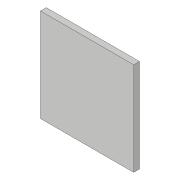
# Autodesk Inventor part: upper part of cappinng system
Saved by Autodesk Inventor 2019 (Build 230136000, 136)
## iProperties
Created: 2019-10-12
Part Number: upper part of cappinng system
Material: Generic
Document SubType Name: Modeling
Designer: Admin
Density: 1 g/cm^3
Appearance: Default
Author: Admin
Autodesk Inventor part; units mm, degrees
ref_plane "YZ Plane" through (0, 0, 0) normal (1, 0, 0) x (0, 1, 0)
ref_plane "XZ Plane" through (0, 0, 0) normal (0, 1, 0) x (-1, 0, 0)
ref_plane "XY Plane" through (0, 0, 0) normal (0, 0, 1) x (1, 0, 0)
sketch "Sketch1" plane through (0, 0, 0) normal (0, 0, 1) x (1, 0, 0)
  line L0 (0, 0) -> (160, 0)
  line L1 (160, 0) -> (160, 160)
  line L2 (160, 160) -> (0, 160)
  line L3 (0, 160) -> (0, 0)
  dimension "d0" = 160
  dimension "d1" = 160
  constraints: 8 end point, 2 parallel, 1 horizontal, 1 perpendicular
  measures "d0" distance of L2.end L1.end
  measures "d1" distance of L1.end L0.end
extrude "Extrusion1" add sketch "Sketch1" along normal blind 10
sketch "Sketch2" plane through (0, 0, 10) normal (0, 0, 1) x (1, 0, 0)
  line L0 (0, 160) -> (0, 0) projected
  line L1 (0, 160) -> (10, 160)
  line L2 (160, 160) -> (0, 160) projected
  line L3 (10, 160) -> (10, 0)
  dimension "d4" = 10
  constraints: 4 end point, 1 perpendicular, 1 point on line
  measures "d4" distance of L0.start L1.end
sketch "Sketch3" plane through (0, 0, 10) normal (0, 0, 1) x (1, 0, 0)
  line L0 (0, 160) -> (0, 0) projected
  line L1 (0, 0) -> (0, 80)
  line L2 (0, 80) -> (159.9334, 80)
  line L3 (0, 0) -> (160, 0) projected
  line L4 (160, 0) -> (150, 0)
  line L5 (150, 0) -> (150, 160)
  line L6 (0, 160) -> (6, 160)
  line L7 (160, 0) -> (160, 160) projected
  line L8 (160, 160) -> (150, 160)
  line L9 (150, 160) -> (150, 150)
  line L10 (150, 150) -> (10, 150)
  line L11 (10, 150) -> (10, 10)
  line L12 (10, 10) -> (150, 10)
  circle A0 centre (10, 150) radius 5
  circle A1 centre (150, 150) radius 5
  circle A2 centre (10, 10) radius 5
  circle A3 centre (150, 10) radius 5
  dimension "d5" = 80
  dimension "d6" = 10
  dimension "d11" = 10
  dimension "d12" = 10
  dimension "d13" = 140
  dimension "d14" = 140
  dimension "d15" = 140
  dimension "d16" = 10
  dimension "d17" = 10
  dimension "d18" = 10
  dimension "d19" = 10
  constraints: 20 end point, 4 centre point, 4 coincident, 4 perpendicular, 3 point on line, 1 horizontal, 1 midpoint
  measures "d5" distance of L0.end L1.end
  measures "d6" distance of L3.end L4.end
  measures "d11" distance of L7.end L5.end
  measures "d12" distance of L5.end L9.end
  measures "d13" distance of L9.end L10.end
  measures "d14" distance of L10.end L11.end
  measures "d15" distance of L11.end L12.end
  measures "d16" diameter of A0
  measures "d17" diameter of A1
  measures "d18" diameter of A2
  measures "d19" diameter of A3
extrude "Extrusion2" [suppressed]
body "Solid1"
